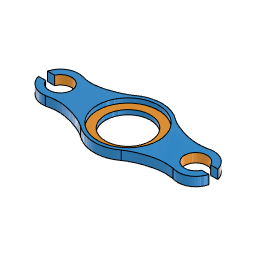
Ex 3 v2 (Autodesk Fusion 360 design; units mm, degrees)
Autodesk Fusion 360 part; units mm, degrees
sketch "Sketch1" plane through (0, 0, 0) normal (0, 0, 1) x (1, 0, 0)
  circle A0 centre (0, 0) radius 50
  circle A1 centre (0, 0) radius 67.8
  line L0 (172.8803, 10.5806) -> (188.6972, 10.6304)
  line L1 (172.9435, -9.4193) -> (188.7603, -9.3695)
  line L2 (-172.9133, 9.9924) -> (-188.7303, 9.9917)
  line L3 (-172.9124, -10.0076) -> (-188.7294, -10.0083)
  arc A2 (172.8803, 10.5806) -> (172.9435, -9.4193) centre (149.9991, 0.5083) ccw
  arc A3 (-172.9124, -10.0076) -> (-172.9133, 9.9924) centre (-150, -0.0066) ccw
  spline S0 degree 5 poles (-142.2948, 39.2444) (-139.5015, 38.696) (-134.0123, 37.1023) (-124.9538, 34.6589) (-109.2698, 34.4162) (-85.3596, 39.9586) (-66.3955, 47.4348) (-54.4735, 53.6359) (-47.933, 57.8567) (-45.0151, 59.9886) knots 0 0 0 0 0 0 0.2 0.4 0.6 0.8 1 1 1 1 1 1
  line L4 (-153.8765, 41.5179) -> (-130.7132, 36.9708)
  line L5 (-52.0796, 54.827) -> (-37.9507, 65.1502)
  spline S1 degree 5 poles (-143.9425, -39.5452) (-141.1288, -39.1142) (-135.5782, -37.7515) (-126.3672, -35.5559) (-110.3854, -35.3011) (-86.0359, -40.4182) (-66.7376, -47.5234) (-54.608, -53.6041) (-47.9536, -57.8445) (-44.9848, -60.0114) knots 0 0 0 0 0 0 0.2 0.4 0.6 0.8 1 1 1 1 1 1
  line L6 (-155.5855, -41.329) -> (-132.2995, -37.7615)
  line L7 (-52.0519, -54.8534) -> (-37.9178, -65.1694)
  spline S2 degree 5 poles (136.9362, 38.3151) (134.2571, 38.1969) (128.9186, 37.5114) (120.0662, 36.2753) (105.0614, 36.7493) (82.6636, 41.8202) (65.0313, 48.4234) (53.9, 54.056) (47.7453, 57.9955) (44.9848, 60.0114) knots 0 0 0 0 0 0 0.2 0.4 0.6 0.8 1 1 1 1 1 1
  line L8 (148.6276, 40.4867) -> (125.1542, 39.4509)
  line L9 (52.0506, 54.8516) -> (37.9191, 65.1712)
  spline S3 degree 5 poles (137.1953, -37.3871) (134.5046, -37.2656) (129.1438, -36.5696) (120.26, -35.3458) (105.2171, -35.9626) (82.7761, -41.3663) (65.1109, -48.2356) (53.955, -53.9918) (47.7839, -57.9668) (45.0152, -59.9886) knots 0 0 0 0 0 0 0.2 0.4 0.6 0.8 1 1 1 1 1 1
  line L10 (148.8626, -39.4812) -> (125.3916, -38.4212)
  line L11 (52.081, -54.8288) -> (37.9495, -65.1484)
  arc A4 (44.9848, 60.0114) -> (-45.0151, 59.9886) centre (0, 0) ccw
  arc A5 (-44.9855, -60.0109) -> (45.0152, -59.9886) centre (0, 0) ccw
  arc A6 (-188.7294, -10.0083) -> (-143.9425, -39.5452) centre (-150, -0.0065) ccw
  arc A7 (-142.2948, 39.2444) -> (-188.7303, 9.9917) centre (-150, -0.0065) ccw
  arc A8 (188.6972, 10.6304) -> (136.9362, 38.3151) centre (149.9991, 0.5083) ccw
  arc A9 (137.1953, -37.3871) -> (188.7603, -9.3695) centre (149.9991, 0.5083) ccw
  dimension "d1" = 100
  dimension "d2" = 135.6
  dimension "d4" = 150
  dimension "d5" = 50
  dimension "d11" = 20
  dimension "d12" = 40
  dimension "d13" = 150
  constraint coincident A0.centre A1.centre
  constraint concentric A0 A4
  constraint concentric A2 A8
  constraint coincident S0.start A6
  constraint coincident S0.end A4
  constraint midpoint S0.start L4
  constraint midpoint S0.end L5
  constraint coincident S1.end A4
  constraint midpoint S1.start L6
  constraint midpoint S1.end L7
  constraint coincident S0 A4.end
  constraint concentric A4 A5
  constraint coincident S1 A5.start
  constraint concentric A6 A7
  constraint concentric A8 A9
  measures "d1" diameter of A0
  measures "d2" diameter of A1
  measures "d4" distance of A0.centre A2.centre
  measures "d5" diameter of A2
  measures "d11" distance of L0 L1
  measures "d12" radius of A9
  measures "d13" distance of A3.centre A0.centre
extrude "Extrude1" add sketch "Sketch1" along normal blind 10 contours A1
extrude "Extrude2" add sketch "Sketch1" along normal blind 20 contours L0 L1 L2 L3 A2 A3 S0 L5 S1 L7 S2 L9 S3 L11 A4 A5 A6 A7 A8 A9 | L9 A4 | L11 A5 | L5 A4 | L7 A5
